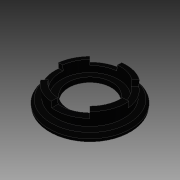
# Autodesk Inventor part: belt_guide
Saved by Autodesk Inventor 2014 (Build 180170000, 170)
## iProperties
Created: 2013-12-02
Part Number: belt_guide
Material: ABS Plastic
Document SubType Name: Modeling
Designer: buben
Density: 1.06 g/cm^3
Appearance: Anodized - Black
Author: buben
Autodesk Inventor part; units mm, degrees
ref_plane "YZ Plane" through (0, 0, 0) normal (1, 0, 0) x (0, 1, 0)
ref_plane "XZ Plane" through (0, 0, 0) normal (0, 1, 0) x (-1, 0, 0)
ref_plane "XY Plane" through (0, 0, 0) normal (0, 0, 1) x (1, 0, 0)
sketch "Sketch1" plane through (0, 0, 0) normal (0, 0, 1) x (1, 0, 0)
  circle A0 centre (0, 0) radius 16
  circle A1 centre (0, 0) radius 8.5
  dimension "d0" = 32
  dimension "d1" = 17
  constraints: 2 centre point, 2 coincident
  measures "d0" diameter of A0
  measures "d1" diameter of A1
extrude "Extrusion1" add sketch "Sketch1" along normal blind 2
sketch "Sketch2" plane through (0, 0, 2) normal (0, 0, 1) x (1, 0, 0)
  circle A0 centre (0, 0) radius 16 projected
  circle A1 centre (0, 0) radius 11
  circle A2 centre (0, 0) radius 13
  dimension "d4" = 22
  dimension "d5" = 26
  constraints: 2 centre point, 2 coincident
  measures "d4" diameter of A1
  measures "d5" diameter of A2
extrude "Extrusion2" add sketch "Sketch2" along normal blind 4.5 contours A2
sketch "Sketch3" plane through (0, 0, 6.5) normal (0, 0, 1) x (1, 0, 0)
  circle A0 centre (0, 0) radius 11 projected
  circle A1 centre (0, 0) radius 13 projected
  line L0 (-13, 0) -> (13, 0) construction
  line L1 (0, 13) -> (0, -13) construction
  line L2 (-9.1924, 9.1924) -> (9.1924, -9.1924) construction
  line L3 (9.1924, 9.1924) -> (-9.1924, -9.1924) construction
  circle A2 centre (0, 0) radius 13
  circle A3 centre (0, 0) radius 11
  line L4 (-13, 0) -> (-11, 0)
  line L5 (-7.7782, 7.7782) -> (-9.1924, 9.1924)
  line L6 (0, 13) -> (0, 11)
  line L7 (7.7782, 7.7782) -> (9.1924, 9.1924)
  line L8 (11, 0) -> (13, 0)
  line L9 (9.1924, -9.1924) -> (7.7782, -7.7782)
  line L10 (0, -11) -> (0, -13)
  line L11 (-7.7782, -7.7782) -> (-9.1924, -9.1924)
  dimension "d8" = 45
  dimension "d9" = 45
  constraints: 24 end point, 9 point on line, 6 midpoint, 4 collinear, 2 coincident, 2 point on circle, 1 centre point, 1 horizontal, 1 perpendicular, 20 other
  measures "d8" angle of L2 L1
  measures "d9" angle of L3 L0
extrude "Extrusion3" cut sketch "Sketch3" against normal blind 2 contours A0 L7 A1 L8 | L9 A1 L10 A0 | A0 L5 A1 L6 | L11 A1 L4 A0
chamfer "Chamfer1" distance 1 angle 45 1 edges at (-16, 0, 2)
body "Solid1"
